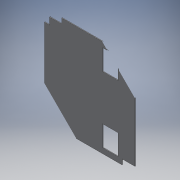
# Autodesk Inventor part: Bellypan
Saved by Autodesk Inventor 2016 (Build 200138000, 138)
## iProperties
Created: 2017-01-08
Part Number: Bellypan
Material: Generic
Document SubType Name: Modeling
Designer: idevr_000
Density: 1 g/cm^3
Appearance: Default
Author: idevr_000
Autodesk Inventor part; units mm, degrees
ref_plane "YZ Plane" through (0, 0, 0) normal (1, 0, 0) x (0, 1, 0)
ref_plane "XZ Plane" through (0, 0, 0) normal (0, 1, 0) x (-1, 0, 0)
ref_plane "XY Plane" through (0, 0, 0) normal (0, 0, 1) x (1, 0, 0)
sketch "Sketch1" plane through (0, 0, 0) normal (0, 0, 1) x (1, 0, 0)
  line L0 (-222.25, -238.125) -> (222.25, -238.125)
  line L1 (222.25, -238.125) -> (222.25, 238.125)
  line L2 (222.25, 238.125) -> (-222.25, 238.125)
  line L3 (-222.25, 238.125) -> (-222.25, -238.125)
  line L4 (-222.25, -238.125) -> (222.25, 238.125) construction
  line L5 (222.25, -238.125) -> (-222.25, 238.125) construction
  point P0 (0, 0)
  dimension "d0" = 444.5
  dimension "d1" = 476.25
  constraints: 12 end point, 2 midpoint, 2 parallel, 1 horizontal, 1 perpendicular
  measures "d0" distance of L2.end L1.end
  measures "d1" distance of L1.end L0.end
extrude "Extrusion1" add sketch "Sketch1" along normal blind 3.175
sketch "Sketch3" plane through (0, 0, 3.175) normal (0, 0, 1) x (1, 0, 0)
  line L0 (-222.25, -238.125) -> (222.25, -238.125) construction
  line L1 (222.25, -238.125) -> (222.25, -161.925) construction
  line L2 (222.25, -238.125) -> (222.25, 238.125) construction
  line L3 (222.25, -161.925) -> (101.6, -161.925) construction
  line L4 (63.5, -212.725) -> (139.7, -212.725)
  line L5 (139.7, -212.725) -> (139.7, -111.125)
  line L6 (139.7, -111.125) -> (63.5, -111.125)
  line L7 (63.5, -111.125) -> (63.5, -212.725)
  line L8 (63.5, -212.725) -> (139.7, -111.125) construction
  line L9 (139.7, -212.725) -> (63.5, -111.125) construction
  point P0 (0, 0)
  dimension "d10" = 76.2
  dimension "d11" = 120.65
  dimension "d12" = 76.2
  dimension "d13" = 101.6
  constraints: 16 end point, 2 midpoint, 2 parallel, 2 perpendicular, 1 horizontal, 1 point on line
  measures "d10" distance of L0.end L1.end
  measures "d11" distance of L1.end L3.end
  measures "d12" distance of L6.end L5.end
  measures "d13" distance of L5.end L4.end
extrude "Extrusion3" cut sketch "Sketch3" against normal through all
sketch "Sketch4" plane through (0, 0, 3.175) normal (0, 0, 1) x (1, 0, 0)
  line L0 (222.25, -238.125) -> (222.25, 238.125) construction
  line L1 (222.25, 238.125) -> (222.25, 161.925) construction
  line L2 (222.25, 161.925) -> (101.6, 161.925) construction
  line L3 (63.5, 111.125) -> (139.7, 111.125)
  line L4 (139.7, 111.125) -> (139.7, 212.725)
  line L5 (139.7, 212.725) -> (63.5, 212.725)
  line L6 (63.5, 212.725) -> (63.5, 111.125)
  line L7 (63.5, 111.125) -> (139.7, 212.725) construction
  line L8 (139.7, 111.125) -> (63.5, 212.725) construction
  point P0 (0, 0)
  dimension "d16" = 76.2
  dimension "d17" = 120.65
  dimension "d18" = 76.2
  dimension "d19" = 101.6
  constraints: 16 end point, 2 midpoint, 2 parallel, 2 perpendicular, 1 horizontal, 1 point on line
  measures "d16" distance of L0.end L1.end
  measures "d17" distance of L1.end L2.end
  measures "d18" distance of L5.end L4.end
  measures "d19" distance of L4.end L3.end
extrude "Extrusion4" cut sketch "Sketch4" against normal through all
sketch "Sketch5" plane through (0, 0, 0) normal (0, 0, -1) x (-1, 0, 0)
  line L0 (-222.25, -238.125) -> (-222.25, 238.125) projected
  line L1 (-222.25, -238.125) -> (-158.75, -238.125)
  line L2 (-158.75, -238.125) -> (-158.75, -212.725)
  line L3 (-158.75, -212.725) -> (-222.25, -212.725)
  line L4 (-222.25, -212.725) -> (-222.25, -238.125)
  point P0 (0, 0)
  dimension "d22" = 63.5
  dimension "d23" = 25.4
  constraints: 8 end point, 2 parallel, 1 horizontal, 1 perpendicular
  measures "d22" distance of L3.end L2.end
  measures "d23" distance of L2.end L1.end
extrude "Extrusion5" cut sketch "Sketch5" against normal through all
sketch "Sketch6" plane through (0, 0, 0) normal (0, 0, -1) x (-1, 0, 0)
  line L0 (-222.25, 238.125) -> (-158.75, 238.125)
  line L1 (-158.75, 238.125) -> (-158.75, 212.725)
  line L2 (-158.75, 212.725) -> (-222.25, 212.725)
  line L3 (-222.25, 212.725) -> (-222.25, 238.125)
  point P0 (0, 0)
  dimension "d26" = 63.5
  dimension "d27" = 25.4
  constraints: 8 end point, 2 parallel, 1 horizontal, 1 perpendicular
  measures "d26" distance of L1.end L2.end
  measures "d27" distance of L0.end L1.end
extrude "Extrusion6" cut sketch "Sketch6" against normal through all
sketch "Sketch7" plane through (0, 0, 0) normal (0, 0, -1) x (-1, 0, 0)
  line L0 (-158.75, 238.125) -> (222.25, 238.125) projected
  line L1 (222.25, 238.125) -> (137.16, 238.125)
  line L2 (137.16, 238.125) -> (137.16, 212.725)
  line L3 (137.16, 212.725) -> (196.85, 212.725)
  line L4 (222.25, 217.4302) -> (222.25, 238.125)
  line L5 (222.25, 238.125) -> (187.6675, 238.125)
  line L6 (196.85, 212.725) -> (196.85, 178.435)
  line L7 (196.85, 178.435) -> (222.25, 178.435)
  line L8 (222.25, 178.435) -> (222.25, 238.125)
  point P0 (0, 0)
  dimension "d31" = 25.4
  dimension "d32" = 25.4
  dimension "d36" = 59.69
  dimension "d37" = 85.09
  constraints: 16 end point, 4 parallel, 2 horizontal, 2 perpendicular
  measures "d31" distance of L2.end L1.end
  measures "d32" distance of L7.end L6.end
  measures "d36" distance between parallel lines of L0 L7
  measures "d37" distance between parallel lines of L8 L2
extrude "Extrusion7" cut sketch "Sketch7" against normal through all
sketch "Sketch8" plane through (0, 0, 0) normal (0, 0, -1) x (-1, 0, 0)
  line L0 (222.25, -238.125) -> (-158.75, -238.125) projected
  line L1 (222.25, -238.125) -> (196.85, -238.125)
  line L2 (196.85, -212.725) -> (196.85, -178.435)
  line L3 (196.85, -178.435) -> (222.25, -178.435)
  line L4 (222.25, -178.435) -> (222.25, -238.125)
  line L5 (222.25, -238.125) -> (137.16, -238.125)
  line L6 (137.16, -238.125) -> (137.16, -212.725)
  line L7 (137.16, -212.725) -> (196.85, -212.725)
  line L8 (222.25, -212.725) -> (222.25, -238.125)
  point P0 (0, 0)
  dimension "d38" = 25.4
  dimension "d39" = 59.69
  dimension "d40" = 85.09
  dimension "d41" = 25.4
  constraints: 16 end point, 4 parallel, 2 horizontal, 2 perpendicular
  measures "d38" distance of L2.end L3.end
  measures "d39" distance of L1.end L2.end
  measures "d40" distance of L6.end L8.start
  measures "d41" distance of L5.end L6.end
extrude "Extrusion8" cut sketch "Sketch8" against normal through all
sketch "Sketch9" plane through (0, 0, 0) normal (0, 0, -1) x (-1, 0, 0)
  line L0 (-158.75, 212.725) -> (-158.75, 238.125) construction
  line L1 (-158.75, 225.425) -> (6.35, 225.425) construction
  line L2 (-50.8, 238.125) -> (63.5, 238.125)
  line L3 (63.5, 238.125) -> (63.5, 212.725)
  line L4 (63.5, 212.725) -> (-50.8, 212.725)
  line L5 (-50.8, 212.725) -> (-50.8, 238.125)
  line L6 (-50.8, 238.125) -> (63.5, 212.725) construction
  line L7 (63.5, 238.125) -> (-50.8, 212.725) construction
  line L8 (-158.75, -238.125) -> (-158.75, -212.725) construction
  line L9 (-158.75, -225.425) -> (6.35, -225.425) construction
  line L10 (-50.8, -212.725) -> (63.5, -212.725)
  line L11 (63.5, -212.725) -> (63.5, -238.125)
  line L12 (63.5, -238.125) -> (-50.8, -238.125)
  line L13 (-50.8, -238.125) -> (-50.8, -212.725)
  line L14 (-50.8, -212.725) -> (63.5, -238.125) construction
  line L15 (63.5, -212.725) -> (-50.8, -238.125) construction
  point P0 (0, 0)
  dimension "d44" = 165.1
  dimension "d45" = 114.3
  dimension "d46" = 25.4
  dimension "d47" = 165.1
  dimension "d48" = 114.3
  dimension "d49" = 25.4
  constraints: 28 end point, 6 midpoint, 4 horizontal, 4 parallel, 2 perpendicular
  measures "d44" distance of L1.start L1.end
  measures "d45" distance of L3.end L4.end
  measures "d46" distance of L2.end L3.end
  measures "d47" distance of L9.start L9.end
  measures "d48" distance of L11.end L12.end
  measures "d49" distance of L10.end L11.end
extrude "Extrusion9" cut sketch "Sketch9" against normal through all
body "Solid1"
